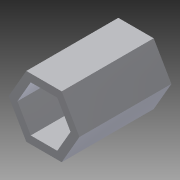
# Autodesk Inventor part: Output Shaft Hex Sleave
Saved by Autodesk Inventor 2013 (Build 170138000, 138)
## iProperties
Created: 2013-06-25
Part Number: Output Shaft Hex Sleave
Material: Generic
Document SubType Name: Modeling
Designer: mvarma
Density: 1 g/cm^3
Author: mvarma
Autodesk Inventor part; units mm, degrees
ref_plane "YZ Plane" through (0, 0, 0) normal (1, 0, 0) x (0, 1, 0)
ref_plane "XZ Plane" through (0, 0, 0) normal (0, 1, 0) x (-1, 0, 0)
ref_plane "XY Plane" through (0, 0, 0) normal (0, 0, 1) x (1, 0, 0)
sketch "Sketch1" plane through (0, 0, 0) normal (0, 0, 1) x (1, 0, 0)
  line L0 (-7.3323, 0) -> (-3.6662, 6.35)
  line L1 (-3.6662, 6.35) -> (3.6662, 6.35)
  line L2 (3.6662, 6.35) -> (7.3323, 0)
  line L3 (7.3323, 0) -> (3.6662, -6.35)
  line L4 (3.6662, -6.35) -> (-3.6662, -6.35)
  line L5 (-3.6662, -6.35) -> (-7.3323, 0)
  line L6 (-2.7496, -4.7625) -> (-5.4993, 0)
  line L7 (-5.4993, 0) -> (-2.7496, 4.7625)
  line L8 (-2.7496, 4.7625) -> (2.7496, 4.7625)
  line L9 (2.7496, 4.7625) -> (5.4993, 0)
  line L10 (5.4993, 0) -> (2.7496, -4.7625)
  line L11 (2.7496, -4.7625) -> (-2.7496, -4.7625)
  point P0 (0, 0)
  point P1 (0, 0)
  point P2 (0, 0)
  dimension "d0" = 12.7
  dimension "d1" = 9.525
  constraints: 24 end point, 2 coincident, 2 horizontal, 26 other
  measures "d0" distance between parallel lines of L4 L1
  measures "d1" distance between parallel lines of L11 L8
extrude "Extrusion1" add sketch "Sketch1" along normal blind 19.05
body "Solid1"
